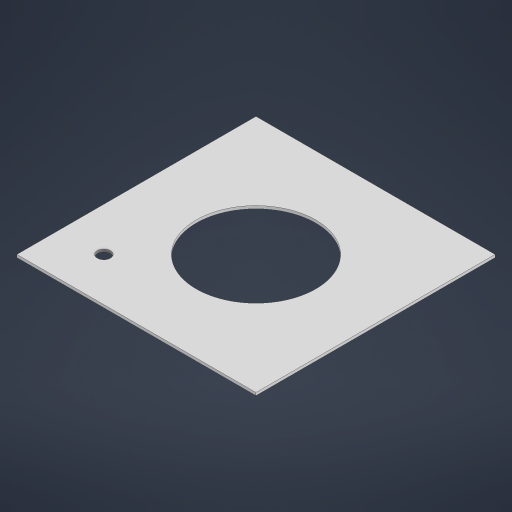
# Autodesk Inventor part: TurretBaseplate
Saved by Autodesk Inventor 2023 (Build 270158000, 158)
## iProperties
Created: 2022-04-16
Part Number: TurretBaseplate
Material: Generic
Document SubType Name: Modeling
Designer: timmy
Density: 1 g/cm^3
Appearance: Default
Author: timmy
Autodesk Inventor part; units mm, degrees
ref_plane "YZ Plane" through (0, 0, 0) normal (1, 0, 0) x (0, 1, 0)
ref_plane "XZ Plane" through (0, 0, 0) normal (0, 1, 0) x (-1, 0, 0)
ref_plane "XY Plane" through (0, 0, 0) normal (0, 0, 1) x (1, 0, 0)
sketch "Sketch1" plane through (0, 0, 0) normal (0, 1, 0) x (-1, 0, 0)
  line L0 (0, 0) -> (279.4, 0)
  line L1 (279.4, 0) -> (279.4, -279.4)
  line L2 (279.4, -279.4) -> (0, -279.4)
  line L3 (0, -279.4) -> (0, 0)
  circle A0 centre (139.7, -139.7) radius 69.85
  dimension "d0" = 279.4
  dimension "d1" = 279.4
  constraints: 8 end point, 2 parallel, 1 centre point, 1 horizontal, 1 perpendicular
  measures "d0" distance of L1.end L2.end
  measures "d1" distance of L0.end L1.end
extrude "Extrusion1" add sketch "Sketch1" along normal blind 3.175
sketch "Sketch3" plane through (0, 3.175, 0) normal (0, 1, 0) x (1, 0, 0)
  line L0 (-279.4, 279.4) -> (-279.4, 0) projected
  line L1 (-279.4, 0) -> (-228.6, 0)
  line L2 (-228.6, 0) -> (-228.6, 50.8)
  line L3 (-228.6, 50.8) -> (-279.4, 50.8)
  line L4 (-279.4, 50.8) -> (-279.4, 0)
  circle A0 centre (-228.6, 50.8) radius 7.62
  point P0 (0, 0)
  dimension "d4" = 50.8
  dimension "d5" = 50.8
  dimension "d6" = 15.24
  constraints: 8 end point, 2 parallel, 1 centre point, 1 coincident, 1 horizontal, 1 perpendicular
  measures "d4" distance of L3.end L2.end
  measures "d5" distance of L2.end L1.end
  measures "d6" diameter of A0
extrude "Extrusion2" cut sketch "Sketch3" against normal blind 3.175 contours A0 L2 L3 | L3 L2 A0
body "Solid1"
